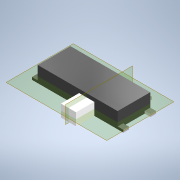
# Autodesk Inventor part: Power Swicth
Saved by Autodesk Inventor 2020 (Build 240168000, 168)
## iProperties
Created: 2021-05-19
Part Number: Power Swicth
Material: Generic
Document SubType Name: Modeling
Designer: Luke
Density: 1 g/cm^3
Appearance: Default
Author: Luke
Autodesk Inventor part; units mm, degrees
ref_plane "YZ Plane" through (0, 0, 0) normal (1, 0, 0) x (0, 1, 0)
ref_plane "XZ Plane" through (0, 0, 0) normal (0, 1, 0) x (-1, 0, 0)
ref_plane "XY Plane" through (0, 0, 0) normal (0, 0, 1) x (1, 0, 0)
sketch "Sketch1" plane through (0, 0, 0) normal (0, 1, 0) x (-1, 0, 0)
  line L0 (-52.5263, -125.0626) -> (-59.1263, -125.0626)
  line L1 (-59.1263, -125.0626) -> (-59.1263, -122.3626)
  line L2 (-59.1263, -122.3626) -> (-52.5263, -122.3626)
  line L3 (-52.5263, -122.3626) -> (-52.5263, -125.0626)
  dimension "d0" = 6.6
  dimension "d1" = 2.7
  constraints: 8 end point, 2 parallel, 1 horizontal, 1 perpendicular
  measures "d0" distance of L1.end L2.end
  measures "d1" distance of L0.end L1.end
extrude "Extrusion1" add sketch "Sketch1" along normal blind 1.3
sketch "Sketch2" plane through (52.5263, 0, -122.3626) normal (0, 0, 1) x (1, 0, 0)
  line L0 (6.6, 0) -> (6.6, 1.3) projected
  line L1 (6.6, 1.3) -> (4.67, 1.3)
  line L2 (0, 1.3) -> (6.6, 1.3) projected
  line L3 (0, 0) -> (6.6, 0) projected
  line L4 (4.67, 0) -> (3.42, 0)
  line L5 (3.42, 0) -> (3.42, 1)
  line L6 (3.42, 1) -> (4.67, 1)
  line L7 (4.67, 1) -> (4.67, 0)
  point P0 (3.42, 0)
  dimension "d4" = 1.93
  dimension "d5" = 1.25
  dimension "d6" = 1
  constraints: 10 end point, 2 parallel, 2 point on line, 1 horizontal, 1 perpendicular
  measures "d4" distance of L0.end L1.end
  measures "d5" distance of L5.end L6.end
  measures "d6" distance of L4.end L5.end
extrude "Extrusion2" add sketch "Sketch2" along normal blind 1.5
sketch "Sketch3" plane through (0, 0, 0) normal (0, -1, 0) x (1, 0, 0)
  line L0 (55.8263, -125.0626) -> (55.8263, -126.2505)
  line L1 (52.5263, -125.0626) -> (52.0463, -125.0626)
  line L2 (52.0463, -125.0626) -> (52.0463, -124.6026)
  line L3 (52.0463, -124.6026) -> (52.5263, -124.6026)
  line L4 (52.5263, -122.3626) -> (52.0463, -122.3626)
  line L5 (52.0463, -122.3626) -> (52.0463, -122.8226)
  line L6 (52.0463, -122.8226) -> (52.5263, -122.8226)
  line L7 (59.1263, -125.0626) -> (59.6063, -125.0626)
  line L8 (59.6063, -125.0626) -> (59.6063, -124.6026)
  line L9 (59.6063, -124.6026) -> (59.1263, -124.6026)
  line L10 (59.1263, -122.3626) -> (59.6063, -122.3626)
  line L11 (59.6063, -122.3626) -> (59.6063, -122.8226)
  line L12 (59.6063, -122.8226) -> (59.1263, -122.8226)
  line L13 (52.5263, -126.3425) -> (53.2263, -126.3425)
  line L14 (59.1263, -125.0626) -> (59.1263, -125.9026)
  line L15 (59.1263, -122.3626) -> (59.1263, -122.8226)
  line L16 (59.1263, -124.6026) -> (59.1263, -125.0626)
  line L17 (52.5263, -125.0626) -> (52.5263, -124.6026)
  line L18 (52.5263, -122.8226) -> (52.5263, -122.3626)
  line L19 (59.1263, -125.0626) -> (52.5263, -125.0626) projected
  line L20 (53.2263, -125.9026) -> (53.6263, -125.9026)
  line L21 (53.6263, -125.9026) -> (53.6263, -125.0626)
  line L22 (53.6263, -125.0626) -> (53.2263, -125.0626)
  line L23 (53.2263, -125.0626) -> (53.2263, -125.9026)
  line L24 (58.4263, -125.9026) -> (58.0263, -125.9026)
  line L25 (58.0263, -125.9026) -> (58.0263, -125.0626)
  line L26 (58.0263, -125.0626) -> (58.4263, -125.0626)
  line L27 (58.4263, -125.0626) -> (58.4263, -125.9026)
  line L28 (58.0263, -125.9026) -> (57.0263, -125.9026)
  line L29 (56.6263, -125.0626) -> (57.0263, -125.0626)
  line L30 (57.0263, -125.0626) -> (57.0263, -125.9026)
  line L31 (56.6263, -125.9026) -> (56.6263, -125.0626)
  line L32 (57.0263, -125.9026) -> (56.6263, -125.9026)
  dimension "d15" = 0.4
  dimension "d16" = 1
  constraints: 64 end point, 11 symmetric about line, 3 horizontal, 2 parallel, 2 perpendicular, 2 point on line, 2 vertical
  measures "d15" distance of L22.end L21.end
  measures "d16" distance of L25.start L28.end
extrude "Extrusion3" add sketch "Sketch3" against normal blind 0.2 contours L1 L2 L3 L17 | L18 L6 L5 L4 | L16 L9 L8 L7 | L10 L11 L12 L15 | L27 L24 L25 L19 | L30 L32 L31 L19 | L21 L20 L23 L19
ref_plane "Work Plane1" through (55.8263, 1.3, -122.3626) normal (1, 0, 0) x (0, 0, -1)
ref_plane "Work Plane2" through (56.5713, 0, -122.3626) normal (-1, 0, 0) x (0, 0, 1)
ref_plane "Work Plane3" through (0, 0.5, 0) normal (0, -1, 0) x (1, 0, 0)
body "Solid1"
